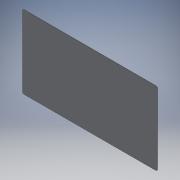
# Autodesk Inventor part: SIde Actylic
Saved by Autodesk Inventor 2019 (Build 230136000, 136)
## iProperties
Created: 2020-07-06
Part Number: SIde Actylic
Material: Generic
Document SubType Name: Modeling
Designer: Vijay
Density: 1 g/cm^3
Appearance: Default
Author: Vijay
Autodesk Inventor part; units mm, degrees
ref_plane "YZ Plane" through (0, 0, 0) normal (1, 0, 0) x (0, 1, 0)
ref_plane "XZ Plane" through (0, 0, 0) normal (0, 1, 0) x (-1, 0, 0)
ref_plane "XY Plane" through (0, 0, 0) normal (0, 0, 1) x (1, 0, 0)
sketch "Sketch1" plane through (0, 0, 0) normal (0, 0, 1) x (1, 0, 0)
  line L0 (-900, -1.9998) -> (-899.9997, -501.9998) projected
  line L1 (100, 28) -> (-900, 28) projected
  line L2 (100, -532) -> (-900, -532) projected
  line L3 (130, -2) -> (130.0002, -502) projected
  line L4 (-890, 28) -> (120.0002, 28)
  line L5 (130.0002, 18) -> (130.0002, -522)
  line L6 (120.0002, -532) -> (-890, -532)
  line L7 (-900, -522) -> (-900, 18)
  arc A0 (-890, 28) -> (-900, 18) centre (-890, 18) ccw
  arc A1 (-900, -522) -> (-890, -532) centre (-890, -522) ccw
  arc A2 (120.0002, -532) -> (130.0002, -522) centre (120.0002, -522) ccw
  arc A3 (130.0002, 18) -> (120.0002, 28) centre (120.0002, 18) ccw
  point P0 (0, 0)
  point P1 (130.0002, -532)
  dimension "d0" = 10
  constraints: 8 end point, 8 point on circle, 8 tangent, 5 point on line, 4 centre point, 3 equal radius, 2 parallel, 1 horizontal, 1 perpendicular
  measures "d0" radius of A0
extrude "Extrusion1" add sketch "Sketch1" along normal blind 3
body "Solid1"
